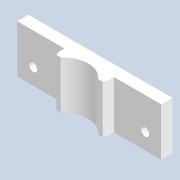
# Autodesk Inventor part: 0008-10-004 Fixare seringa
Saved by Autodesk Inventor 2020 (Build 240168000, 168)
## iProperties
Created: 2021-02-22
Part Number: 0008-10-004 Fixare seringa
Material: ABS Plastic
Document SubType Name: Modeling
Designer: Iulian Bors
Density: 1.06 g/cm^3
Appearance: Smooth - White
Mass: 14.1067 g
Surface Area: 54.8528 cm^2
Volume: 13.3082 cm^3
Description: Fixare Seringa
Author: Iulian Bors
Subject: 004
Autodesk Inventor part; units mm, degrees
ref_plane "YZ Plane" through (0, 0, 0) normal (1, 0, 0) x (0, 1, 0)
ref_plane "XZ Plane" through (0, 0, 0) normal (0, 1, 0) x (-1, 0, 0)
ref_plane "XY Plane" through (0, 0, 0) normal (0, 0, 1) x (1, 0, 0)
sketch "Sketch1" plane through (0, 0, 0) normal (0, 0, 1) x (1, 0, 0)
  line L0 (-45, 10) -> (45, 10)
  line L1 (45, 10) -> (45, -10)
  line L2 (45, -10) -> (-45, -10)
  line L3 (-45, -10) -> (-45, 10)
  point P0 (0, 0)
  point P1 (0, 10)
  point P2 (-45, 0)
  dimension "d0" = 20
  dimension "d1" = 90
  constraints: 8 end point, 2 midpoint, 2 parallel, 1 horizontal, 1 horizontal alignment, 1 perpendicular, 1 vertical alignment
  measures "d0" distance of L2.end L0.start
  measures "d1" distance of L0.start L0.end
extrude "Extrusion1" add sketch "Sketch1" along normal blind 13
sketch "Sketch3" plane through (-45, 10, 0) normal (0, 1, 0) x (1, 0, 0)
  line L0 (90, 0) -> (90, -13) projected
  line L1 (90, -13) -> (0, -13) projected
  line L2 (90, -13) -> (60.5, -13)
  line L3 (60.5, -13) -> (60.5, -7)
  line L4 (60.5, -7) -> (90, -7)
  line L5 (90, -7) -> (90, -13)
  point P0 (45, 0)
  point P1 (60.5, -13)
  dimension "d8" = 6
  dimension "d20" = 15.5
  constraints: 8 end point, 2 collinear, 2 parallel, 1 horizontal, 1 perpendicular
  measures "d8" distance between parallel lines of L1 L4
  measures "d20" distance from line of L3 point (45, 0)
extrude "Extrusion2" cut sketch "Sketch3" against normal through all
mirror "Mirror1" about plane through (0, 0, 0) normal (1, 0, 0) of "Extrusion2"
sketch "Sketch4" plane through (-45, 10, 0) normal (0, 1, 0) x (1, 0, 0)
  line L0 (42, -26.343) -> (42, -14.343)
  line L1 (48, -22.843) -> (48, -17.843)
  line L2 (45, -24.843) -> (45, -15.843)
  line L3 (39, -27.343) -> (39, -13.343)
  line L4 (8, -14.343) -> (8, -26.343)
  line L5 (11, -13.343) -> (11, -27.343)
  line L6 (5, -15.843) -> (5, -24.843)
  line L7 (2, -17.843) -> (2, -22.843)
  circle A0 centre (45, -23.343) radius 15.65
  line L8 (90, 0) -> (0, 0) projected
  point P0 (45, 0)
  point P1 (45, 0)
  dimension "d21" = 31.3
  dimension "d22" = 23.343
  constraints: 16 end point, 8 vertical, 1 centre point, 1 midpoint, 1 vertical alignment, 16 other
  measures "d21" diameter of A0
  measures "d22" distance from line of L8 A0.centre
extrude "Extrusion3" cut sketch "Sketch4" against normal through all
chamfer "Chamfer1" distance 1 distance2 3 1 edges at (-15.5, 0, 13) measured on face at (-12.9967, 3.3333, 13)
chamfer "Chamfer2" distance 1 distance2 3 1 edges at (15.5, 0, 13) measured on face at (14.2483, -3.3333, 13)
sketch "Sketch5" plane through (0, 0, 0) normal (0, 0, -1) x (-1, 0, 0)
  line L0 (45, -10) -> (-45, -10) projected
  line L1 (0, 23.0048) -> (0, -23.0048) construction
  point P0 (0, 0)
  point P1 (-35, 0)
  point P2 (35, 0)
  point P3 (0, 0)
  dimension "d23" = 70
  constraints: 3 horizontal alignment, 2 end point, 1 coincident, 1 midpoint, 1 symmetric about line, 1 vertical
  measures "d23" distance of point (35, 0) point (-35, 0)
hole "Hole1" at (35, 0, 0) at (-35, 0, 0) direction (0, 0, 1) diameter 5 end through all
sketch "Sketch6" plane through (-45, 10, 0) normal (0, 1, 0) x (1, 0, 0)
  line L0 (60.5, -10) -> (59.5, -13) projected
  line L1 (60.5, -10) -> (60.5, -7) projected
  line L2 (60.5, -7) -> (90, -7) projected
  line L3 (90, 0) -> (90, -7) projected
  line L4 (90, 0) -> (0, 0) projected
  line L5 (0, 0) -> (0, -7) projected
  line L6 (0, -7) -> (29.5, -7) projected
  line L7 (29.5, -7) -> (29.5, -10) projected
  line L8 (30.5, -13) -> (29.5, -10) projected
  line L9 (33.255, -13) -> (30.5, -13) projected
  arc A0 (56.745, -13) -> (33.255, -13) centre (45, -23.343) ccw projected
  line L10 (59.5, -13) -> (56.745, -13) projected
  line L11 (60.5, -7) -> (60.5, 0)
  line L12 (90, 0) -> (0, 0) projected
  line L13 (29.5, -7) -> (29.5, 0)
  line L14 (0, 0) -> (90, 0) projected
  point P0 (45, 0)
  constraints: 4 end point, 2 point on line, 1 collinear, 1 perpendicular
extrude "Extrusion4" add sketch "Sketch6" along normal blind 10
sketch "Sketch7" plane through (-45, -10, 7) normal (0, 0, 1) x (1, 0, 0)
  line L0 (29.5, 23.5) -> (60.5, 23.5)
  line L1 (60.5, 23.5) -> (60.5, 20)
  line L2 (60.5, 20) -> (29.5, 20)
  line L3 (29.5, 20) -> (29.5, 23.5)
  line L4 (13, 20) -> (27.9, 20)
  line L5 (90, 30) -> (0, 30) projected
  line L6 (60.5, 30) -> (60.5, 0) projected
  point P0 (45, 10)
  point P1 (45, 23.5)
  point P2 (45, 30)
  dimension "d33" = 3.5
  constraints: 10 end point, 2 collinear, 2 horizontal, 2 midpoint, 2 parallel, 1 perpendicular, 1 vertical alignment, 2 other
  measures "d33" distance of L2.end L0.start
extrude "Extrusion5" cut sketch "Sketch7" against normal through all both and the other way through all
body "Solid1"
